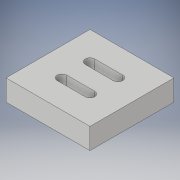
# Autodesk Inventor part: slotted riser 1
Saved by Autodesk Inventor 2019 (Build 230136000, 136)
## iProperties
Created: 2019-04-23
Part Number: slotted riser 1
Material: Generic
Document SubType Name: Modeling
Designer: dewanlab
Density: 1 g/cm^3
Appearance: Default
Author: dewanlab
Autodesk Inventor part; units mm, degrees
ref_plane "YZ Plane" through (0, 0, 0) normal (1, 0, 0) x (0, 1, 0)
ref_plane "XZ Plane" through (0, 0, 0) normal (0, 1, 0) x (-1, 0, 0)
ref_plane "XY Plane" through (0, 0, 0) normal (0, 0, 1) x (1, 0, 0)
sketch "Sketch1" plane through (0, 0, 0) normal (0, 1, 0) x (-1, 0, 0)
  line L0 (21.4105, 40.3607) -> (-54.7895, 40.3607)
  line L1 (-54.7895, 40.3607) -> (-54.7895, -35.8393)
  line L2 (-54.7895, -35.8393) -> (21.4105, -35.8393)
  line L3 (21.4105, -35.8393) -> (21.4105, 40.3607)
  point P0 (0, 0)
  dimension "d0" = 76.2
  dimension "d1" = 76.2
  constraints: 8 end point, 2 parallel, 1 horizontal, 1 perpendicular
  measures "d0" distance of L2.end L0.start
  measures "d1" distance of L1.end L2.end
extrude "Extrusion1" add sketch "Sketch1" along normal blind 19.05
sketch "Sketch2" plane through (0, 19.05, 0) normal (0, 1, 0) x (1, 0, 0)
  arc A0 (3.9895, -10.6427) -> (3.9895, -19.2787) centre (3.9895, -14.9607) ccw
  line L0 (-21.4105, 35.8393) -> (-21.4105, -40.3607) projected
  line L1 (-21.4105, -40.3607) -> (54.7895, -40.3607) projected
  arc A1 (29.3895, -19.2787) -> (29.3895, -10.6427) centre (29.3895, -14.9607) ccw
  line L2 (54.7895, -40.3607) -> (54.7895, 35.8393) projected
  line L3 (3.9895, -19.2787) -> (29.3895, -19.2787)
  line L4 (3.9895, -10.6427) -> (29.3895, -10.6427)
  point P0 (0, 0)
  dimension "d4" = 8.636
  dimension "d5" = 25.4
  dimension "d6" = 25.4
  dimension "d7" = 8.636
  dimension "d8" = 25.4
  dimension "d9" = 25.4
  constraints: 4 end point, 4 point on circle, 2 centre point, 2 tangent
  measures "d4" diameter of A0
  measures "d5" distance from line of L0 A0.centre
  measures "d6" distance from line of A0.centre L1
  measures "d7" diameter of A1
  measures "d8" distance from line of L1 A1.centre
  measures "d9" distance from line of L2 A1.centre
extrude "Extrusion2" cut sketch "Sketch2" against normal through all
sketch "Sketch3" plane through (0, 19.05, 0) normal (0, 1, 0) x (1, 0, 0)
  arc A0 (3.9895, 14.7573) -> (3.9895, 6.1213) centre (3.9895, 10.4393) ccw
  line L0 (-21.4105, 35.8393) -> (-21.4105, -40.3607) projected
  line L1 (54.7895, 35.8393) -> (-21.4105, 35.8393) projected
  arc A1 (29.3895, 6.1213) -> (29.3895, 14.7573) centre (29.3895, 10.4393) ccw
  line L2 (54.7895, -40.3607) -> (54.7895, 35.8393) projected
  line L3 (3.9895, 6.1213) -> (29.3895, 6.1213)
  line L4 (3.9895, 14.7573) -> (29.3895, 14.7573)
  point P0 (0, 0)
  dimension "d12" = 8.636
  dimension "d13" = 25.4
  dimension "d14" = 25.4
  dimension "d15" = 8.636
  dimension "d16" = 25.4
  dimension "d17" = 25.4
  constraints: 4 end point, 4 point on circle, 2 centre point, 2 tangent
  measures "d12" diameter of A0
  measures "d13" distance from line of L0 A0.centre
  measures "d14" distance from line of L1 A0.centre
  measures "d15" diameter of A1
  measures "d16" distance from line of L1 A1.centre
  measures "d17" distance from line of L2 A1.centre
extrude "Extrusion3" add sketch "Sketch3" against normal through all
sketch "Sketch4" plane through (0, 19.05, 0) normal (0, 1, 0) x (1, 0, 0)
  arc A0 (3.9895, 14.7573) -> (3.9895, 6.1213) centre (3.9895, 10.4393) ccw
  line L0 (54.7895, 35.8393) -> (-21.4105, 35.8393) projected
  line L1 (-21.4105, 35.8393) -> (-21.4105, -40.3607) projected
  arc A1 (29.3895, 6.1213) -> (29.3895, 14.7573) centre (29.3895, 10.4393) ccw
  line L2 (54.7895, -40.3607) -> (54.7895, 35.8393) projected
  line L3 (3.9895, 6.1213) -> (29.3895, 6.1213)
  line L4 (29.3895, 14.7573) -> (3.9895, 14.7573)
  point P0 (0, 0)
  dimension "d20" = 8.636
  dimension "d21" = 25.4
  dimension "d22" = 25.4
  dimension "d23" = 8.636
  dimension "d24" = 25.4
  dimension "d25" = 25.4
  constraints: 4 end point, 4 point on circle, 3 tangent, 2 centre point
  measures "d20" diameter of A0
  measures "d21" distance from line of L0 A0.centre
  measures "d22" distance from line of L1 A0.centre
  measures "d23" diameter of A1
  measures "d24" distance from line of L0 A1.centre
  measures "d25" distance from line of L2 A1.centre
extrude "Extrusion4" cut sketch "Sketch4" against normal blind 19.05
body "Solid1"
